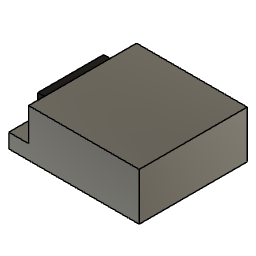
assembly_well plate track v43 (Autodesk Fusion 360 archive; units mm, degrees)
design "meanwell rd-35"
Autodesk Fusion 360 part; units mm, degrees
note: some values were not read from the file. Set by a fixed rule: the direction of a hole.
(part 1 of 2)
sketch "Sketch1" plane through (0, 0, 0) normal (0, 0, 1) x (1, 0, 0)
  line L0 (49.5, -41) -> (-49.5, -41)
  line L1 (-49.5, -41) -> (-49.5, 41)
  line L2 (-49.5, 41) -> (49.5, 41)
  line L3 (49.5, 41) -> (49.5, -41)
  line L4 (49.5, -41) -> (-49.5, 41) construction
  line L5 (-49.5, -41) -> (49.5, 41) construction
  line L6 (-29, -0.5) -> (26, -0.5)
  dimension "d1" = 99
  dimension "d2" = 82
  dimension "d3" = 40.5
  dimension "d4" = 20.5
  dimension "d5" = 55
  constraint horizontal L0
  constraint perpendicular L0 L1
  constraint parallel L0 L2
  constraint parallel L1 L3
  constraint coincident L4 origin
  constraint coincident L5 origin
  constraint horizontal L6
  measures "d1" distance of L1.end L2.end
  measures "d2" distance of L0.end L1.end
  measures "d3" distance of L0 L6
  measures "d4" distance of L1 L6.start
  measures "d5" distance of L6.start L6.end
extrude "Extrude1" add sketch "Sketch1" along normal blind 36 makes body 1
hole "Hole1" at (-29, -0.5, 0) at (26, -0.5, 0) direction (0, 0, 1) diameter 3 depth 10 tip angle 180 bodies 1
sketch "Sketch2" plane through (0, 0, 36) normal (0, 0, 1) x (-1, 0, 0)
  line L0 (-49.5, -41) -> (49.5, -41)
  line L1 (49.5, -41) -> (49.5, 41)
  line L2 (49.5, 41) -> (-49.5, 41)
  line L3 (-49.5, 41) -> (-49.5, -41)
  line L4 (49.5, -41) -> (34.5, -41)
  line L5 (34.5, -41) -> (34.5, 41)
  line L6 (34.5, 41) -> (49.5, 41)
  line L7 (49.5, 41) -> (49.5, -41)
  dimension "d11" = 15
  constraint horizontal L4
  constraint vertical L5
  constraint horizontal L6
  constraint vertical L7
  constraint coincident L2 L5.end
  constraint coincident L0.end L1.start
  measures "d11" distance of L0.end L4.end
extrude "Extrude2" cut sketch "Sketch2" against normal blind 25 contours L0 L1 L2 L4 L5 L6 L7 bodies 1
sketch "Sketch3" plane through (0, 0, 11) normal (0, 0, 1) x (-1, 0, 0)
  line L0 (49.5, 41) -> (34.5, 41)
  line L1 (34.5, 41) -> (34.5, -41)
  line L2 (34.5, -41) -> (49.5, -41)
  line L3 (49.5, -41) -> (49.5, 41)
  line L4 (49.5, -31) -> (34.5, -31)
  line L5 (34.5, -31) -> (34.5, 19)
  line L6 (34.5, 19) -> (49.5, 19)
  line L7 (49.5, 19) -> (49.5, -31)
  dimension "d14" = 10
  dimension "d15" = 50
  constraint horizontal L4
  constraint vertical L5
  constraint horizontal L6
  constraint vertical L7
  constraint coincident L1 L5.end
  constraint coincident L3 L4.start
  measures "d14" distance of L2 L4
  measures "d15" distance of L4.start L6.end
extrude "Extrude3" add sketch "Sketch3" along normal blind 15 separate body contours L1 L3 L4 L5 L6 L7 makes body 2

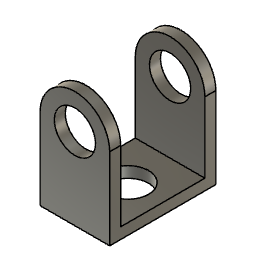
design "actuonix mounting bracket"
Autodesk Fusion 360 part; units mm, degrees
sketch "Sketch1" plane through (0, 0, 0) normal (0, 0, 1) x (1, 0, 0)
  line L0 (3.8, 5.8) -> (-3.8, 5.8)
  line L1 (-3.8, 5.8) -> (-3.8, -5.8)
  line L2 (-3.8, -5.8) -> (3.8, -5.8)
  line L3 (3.8, -5.8) -> (3.8, 5.8)
  line L4 (3.8, 5.8) -> (-3.8, -5.8) construction
  line L5 (-3.8, 5.8) -> (3.8, -5.8) construction
  dimension "d1" = 7.6
  dimension "d2" = 11.6
  constraint horizontal L0
  constraint perpendicular L0 L1
  constraint parallel L0 L2
  constraint parallel L1 L3
  constraint coincident L4 origin
  constraint coincident L5 origin
  measures "d1" distance of L0.start L0.end
  measures "d2" distance of L0.end L1.end
extrude "Extrude1" add sketch "Sketch1" along normal blind 12.7
sketch "Sketch2" plane through (3.8, 0, 0) normal (1, 0, 0) x (0, 1, 0)
  line L0 (-5.8, 0) -> (5.8, 0)
  line L1 (5.8, 0) -> (5.8, 12.7)
  line L2 (5.8, 12.7) -> (-5.8, 12.7)
  line L3 (-5.8, 12.7) -> (-5.8, 0)
  line L4 (-4.6, 11.5) -> (-4.6, 1.2)
  line L5 (-4.6, 1.2) -> (4.6, 1.2)
  line L6 (4.6, 1.2) -> (4.6, 11.5)
  line L7 (4.6, 11.5) -> (-4.6, 11.5)
  line L8 (4.6, 11.5) -> (4.6, 12.7)
  line L9 (-4.6, 11.5) -> (-4.6, 12.7)
  dimension "d5" = -1.2
  constraint coincident L2 L8.end
  constraint perpendicular L2 L8
  constraint coincident L2 L9.end
  constraint perpendicular L2 L9
extrude "Extrude2" cut sketch "Sketch2" against normal up to surface (7.6 mm away) contours L2 L7 L8 L9 | L4 L5 L6 L7
fillet "Fillet1" radius 3.8 4 edges at (3.8, 5.2, 12.7) (-3.8, 5.2, 12.7) (3.8, -5.2, 12.7) (-3.8, -5.2, 12.7)
hole "Hole1" at (0, 5.8, 8.9) direction (0, -1, 0) diameter 4.5 end through all
hole "Hole2" at (0, 0, 1.2) direction (0, 0, -1) diameter 4.5 end through all
equation "d9 = ( 7.6 / 2 ) * 1 mm"

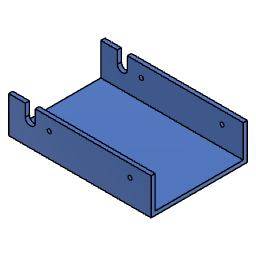
design "moving tray"
Autodesk Fusion 360 part; units mm, degrees
sketch "Sketch1" plane through (0, 0, 0) normal (0, 0, 1) x (1, 0, 0)
  line L0 (107.5, -72.5) -> (-107.5, -72.5)
  line L1 (-107.5, -72.5) -> (-107.5, 72.5)
  line L2 (-107.5, 72.5) -> (107.5, 72.5)
  line L3 (107.5, 72.5) -> (107.5, -72.5)
  line L4 (107.5, -72.5) -> (-107.5, 72.5) construction
  line L5 (-107.5, -72.5) -> (107.5, 72.5) construction
  dimension "d1" = 215
  dimension "d2" = 145
  constraint horizontal L0
  constraint perpendicular L0 L1
  constraint parallel L0 L2
  constraint parallel L1 L3
  constraint coincident L4 origin
  constraint coincident L5 origin
  measures "d1" distance of L1.end L2.end
  measures "d2" distance of L0.end L1.end
extrude "Extrude1" add sketch "Sketch1" along normal blind 55
sketch "Sketch2" plane through (-107.5, 0, 0) normal (-1, 0, 0) x (0, -1, 0)
  line L0 (-72.5, 0) -> (72.5, 0)
  line L1 (72.5, 0) -> (72.5, 55)
  line L2 (72.5, 55) -> (-72.5, 55)
  line L3 (-72.5, 55) -> (-72.5, 0)
  line L4 (-66.5, 49) -> (-66.5, 6)
  line L5 (-66.5, 6) -> (66.5, 6)
  line L6 (66.5, 6) -> (66.5, 49)
  line L7 (66.5, 49) -> (-66.5, 49)
  line L8 (66.5, 49) -> (66.5, 55)
  line L9 (-66.5, 49) -> (-66.5, 55)
  dimension "d5" = -6
  constraint coincident L2 L8.end
  constraint perpendicular L2 L8
  constraint coincident L2 L9.end
  constraint perpendicular L2 L9
extrude "Extrude2" cut sketch "Sketch2" against normal through all contours L2 L7 L8 L9 | L4 L5 L6 L7
sketch "Sketch3" plane through (0, 72.5, 0) normal (0, 1, 0) x (-1, 0, 0)
  line L0 (-107.5, 0) -> (107.5, 0)
  line L1 (107.5, 0) -> (107.5, 55)
  line L2 (107.5, 55) -> (-107.5, 55)
  line L3 (-107.5, 55) -> (-107.5, 0)
  line L4 (107.5, 6) -> (107.5, 55)
  line L5 (107.5, 36.5) -> (46.5, 36.5)
  line L6 (46.5, 36.5) -> (-75.5, 36.5)
  point P0 (46.5, 36.5)
  dimension "d7" = 122
  dimension "d8" = 61
  dimension "d9" = 18.5
  constraint perpendicular L1 L5
  constraint perpendicular L1 L6
  constraint coincident L4 L5.start
  constraint coincident P0 L5.end
  measures "d7" distance of P0 L6.end
  measures "d8" distance of L5.start P0
  measures "d9" distance of L2 L5
hole "Hole1" at (-46.5, 72.5, 36.5) at (75.5, 72.5, 36.5) direction (0, -1, 0) diameter 5.944 end through all
sketch "Sketch4" plane through (0, -72.5, 0) normal (0, -1, 0) x (1, 0, 0)
  circle A0 centre (-46.5, 36.5) radius 2.972
  circle A1 centre (75.5, 36.5) radius 2.972
  line L0 (-107.5, 0) -> (107.5, 0)
  line L1 (107.5, 0) -> (107.5, 55)
  line L2 (107.5, 55) -> (-107.5, 55)
  line L3 (-107.5, 55) -> (-107.5, 0)
  circle A2 centre (-75, 36.5) radius 7.5
  line L4 (-67.5, 36.5) -> (-67.5, 55)
  line L5 (-82.5, 36.5) -> (-82.5, 55)
  dimension "d13" = 28.5
  dimension "d14" = 15
  constraint horizontal A0.centre A2.centre
  constraint coincident A2 L4.start
  constraint coincident L2 L4.end
  constraint tangent A2 L4
  constraint coincident A2 L5.start
  constraint coincident L2 L5.end
  constraint tangent A2 L5
  constraint vertical L5
  constraint vertical L4
  measures "d13" distance of A0.centre A2.centre
  measures "d14" diameter of A2
extrude "Extrude3" cut sketch "Sketch4" against normal through all contours L2 A2 L4 L5 | A2

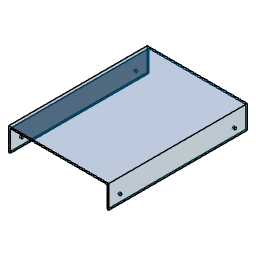
design "well plate base"
Autodesk Fusion 360 part; units mm, degrees
sketch "Sketch1" plane through (0, 0, 0) normal (0, 0, 1) x (1, 0, 0)
  line L0 (65, 90) -> (-65, 90)
  line L1 (-65, 90) -> (-65, -90)
  line L2 (-65, -90) -> (65, -90)
  line L3 (65, -90) -> (65, 90)
  line L4 (65, 90) -> (-65, -90) construction
  line L5 (-65, 90) -> (65, -90) construction
  dimension "d1" = 130
  dimension "d2" = 180
  constraint horizontal L0
  constraint perpendicular L0 L1
  constraint parallel L0 L2
  constraint parallel L1 L3
  constraint coincident L4 origin
  constraint coincident L5 origin
  measures "d1" distance of L1.end L2.end
  measures "d2" distance of L0.end L1.end
extrude "Extrude1" add sketch "Sketch1" along normal blind 30
shell "Shell1" thickness 2 removed faces 1 at (21.6667, -30, 0)
sketch "Sketch3" plane through (0, -90, 0) normal (0, -1, 0) x (1, 0, 0)
  line L0 (-65, 0) -> (65, 0)
  line L1 (65, 0) -> (65, 30)
  line L2 (65, 30) -> (-65, 30)
  line L3 (-65, 30) -> (-65, 0)
  line L4 (-63, 28) -> (63, 28)
  line L5 (63, 28) -> (63, 0)
  line L6 (63, 0) -> (-63, 0)
  line L7 (-63, 0) -> (-63, 28)
  point P0 (-63, 28)
  point P1 (63, 0)
  constraint horizontal L4
  constraint vertical L5
  constraint horizontal L6
  constraint vertical L7
  constraint coincident P1 L5.end
  constraint coincident P0 L4.start
extrude "Extrude3" cut sketch "Sketch3" against normal through all contours L0 L4 L5 L6 L7
sketch "Sketch4" plane through (65, 0, 0) normal (1, 0, 0) x (0, 1, 0)
  line L0 (-90, 0) -> (90, 0)
  line L1 (90, 0) -> (90, 30)
  line L2 (90, 30) -> (-90, 30)
  line L3 (-90, 30) -> (-90, 0)
  line L4 (-74.25, 10) -> (74.25, 10)
  line L5 (0, 0) -> (0, 10)
  dimension "d9" = 148.5
  dimension "d10" = 10
  constraint parallel L2 L4
  constraint coincident L5.start origin
  constraint coincident L4 L5.end
  constraint midpoint L4 L5.end
  constraint vertical L5
  measures "d9" distance of L4.start L4.end
  measures "d10" distance of L0 L4
hole "Hole1" at (65, -74.25, 10) at (65, 74.25, 10) direction (-1, 0, 0) diameter 3 depth 164 tip angle 118

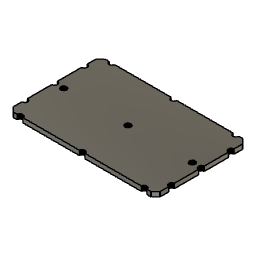
design "solderful protoboard"
Autodesk Fusion 360 part; units mm, degrees
sketch "SOLDERBREAD02_DXF_Outline_in_MilliMeters" plane through (0, 0, 0) normal (0, 0, 1) x (1, 0, 0)
  line L0 (116.847, -64.0665) -> (116.619, -64.1211)
  line L1 (116.619, -64.1211) -> (116.403, -64.2106)
  line L2 (116.403, -64.2106) -> (116.204, -64.3328)
  line L3 (116.204, -64.3328) -> (116.026, -64.4848)
  line L4 (116.026, -64.4848) -> (115.874, -64.6627)
  line L5 (115.874, -64.6627) -> (115.752, -64.8621)
  line L6 (115.752, -64.8621) -> (115.662, -65.0783)
  line L7 (115.662, -65.0783) -> (115.607, -65.3058)
  line L8 (115.607, -65.3058) -> (115.589, -65.539)
  line L9 (115.589, -65.539) -> (115.607, -65.7722)
  line L10 (115.607, -65.7722) -> (115.662, -65.9997)
  line L11 (115.662, -65.9997) -> (115.752, -66.2159)
  line L12 (115.752, -66.2159) -> (115.874, -66.4153)
  line L13 (115.874, -66.4153) -> (116.026, -66.5932)
  line L14 (116.026, -66.5932) -> (116.204, -66.7452)
  line L15 (116.204, -66.7452) -> (116.403, -66.8674)
  line L16 (116.403, -66.8674) -> (116.619, -66.9569)
  line L17 (116.619, -66.9569) -> (116.847, -67.0115)
  line L18 (116.847, -67.0115) -> (117.071, -67.0292)
  line L19 (117.071, -67.0292) -> (117.08, -67.0253)
  line L20 (117.08, -67.0253) -> (117.098, -67.0326)
  line L21 (117.098, -67.0326) -> (117.105, -67.0503)
  line L22 (117.105, -67.0503) -> (117.105, -80.511)
  line L23 (117.105, -80.511) -> (117.098, -80.5287)
  line L24 (117.098, -80.5287) -> (117.08, -80.536)
  line L25 (117.08, -80.536) -> (117.068, -80.531)
  line L26 (117.068, -80.531) -> (116.842, -80.5488)
  line L27 (116.842, -80.5488) -> (116.611, -80.6044)
  line L28 (116.611, -80.6044) -> (116.39, -80.6956)
  line L29 (116.39, -80.6956) -> (116.187, -80.8202)
  line L30 (116.187, -80.8202) -> (116.006, -80.975)
  line L31 (116.006, -80.975) -> (115.851, -81.1562)
  line L32 (115.851, -81.1562) -> (115.727, -81.3594)
  line L33 (115.727, -81.3594) -> (115.635, -81.5796)
  line L34 (115.635, -81.5796) -> (115.58, -81.8114)
  line L35 (115.58, -81.8114) -> (115.561, -82.049)
  line L36 (115.561, -82.049) -> (115.58, -82.2866)
  line L37 (115.58, -82.2866) -> (115.635, -82.5184)
  line L38 (115.635, -82.5184) -> (115.727, -82.7386)
  line L39 (115.727, -82.7386) -> (115.851, -82.9418)
  line L40 (115.851, -82.9418) -> (116.006, -83.123)
  line L41 (116.006, -83.123) -> (116.187, -83.2778)
  line L42 (116.187, -83.2778) -> (116.39, -83.4024)
  line L43 (116.39, -83.4024) -> (116.611, -83.4936)
  line L44 (116.611, -83.4936) -> (116.842, -83.5492)
  line L45 (116.842, -83.5492) -> (117.07, -83.5671)
  line L46 (117.07, -83.5671) -> (117.08, -83.563)
  line L47 (117.08, -83.563) -> (117.098, -83.5703)
  line L48 (117.098, -83.5703) -> (117.105, -83.588)
  line L49 (117.105, -83.588) -> (117.105, -88.233)
  line L50 (117.105, -88.233) -> (117.105, -88.2333)
  line L51 (117.105, -88.2333) -> (117.105, -88.2336)
  line L52 (117.105, -88.2336) -> (117.105, -88.2336)
  line L53 (117.105, -88.2336) -> (117.098, -88.3175)
  line L54 (117.098, -88.3175) -> (117.073, -88.3981)
  line L55 (117.073, -88.3981) -> (117.033, -88.4721)
  line L56 (117.033, -88.4721) -> (116.979, -88.535)
  line L57 (116.979, -88.535) -> (116.979, -88.5357)
  line L58 (116.979, -88.5357) -> (114.679, -90.8352)
  line L59 (114.679, -90.8352) -> (114.678, -90.8356)
  line L60 (114.678, -90.8356) -> (114.616, -90.8902)
  line L61 (114.616, -90.8902) -> (114.542, -90.9313)
  line L62 (114.542, -90.9313) -> (114.461, -90.9563)
  line L63 (114.461, -90.9563) -> (114.377, -90.964)
  line L64 (114.377, -90.964) -> (114.377, -90.964)
  line L65 (114.377, -90.964) -> (114.376, -90.9636)
  line L66 (114.376, -90.9636) -> (114.375, -90.964)
  line L67 (114.375, -90.964) -> (112.259, -90.964)
  line L68 (112.259, -90.964) -> (112.241, -90.9567)
  line L69 (112.241, -90.9567) -> (112.234, -90.939)
  line L70 (112.234, -90.939) -> (112.238, -90.9297)
  line L71 (112.238, -90.9297) -> (112.22, -90.7074)
  line L72 (112.22, -90.7074) -> (112.166, -90.4814)
  line L73 (112.166, -90.4814) -> (112.077, -90.2668)
  line L74 (112.077, -90.2668) -> (111.956, -90.0687)
  line L75 (111.956, -90.0687) -> (111.805, -89.892)
  line L76 (111.805, -89.892) -> (111.628, -89.7411)
  line L77 (111.628, -89.7411) -> (111.43, -89.6197)
  line L78 (111.43, -89.6197) -> (111.216, -89.5308)
  line L79 (111.216, -89.5308) -> (110.99, -89.4765)
  line L80 (110.99, -89.4765) -> (110.758, -89.4583)
  line L81 (110.758, -89.4583) -> (110.526, -89.4765)
  line L82 (110.526, -89.4765) -> (110.3, -89.5308)
  line L83 (110.3, -89.5308) -> (110.086, -89.6197)
  line L84 (110.086, -89.6197) -> (109.888, -89.7411)
  line L85 (109.888, -89.7411) -> (109.711, -89.892)
  line L86 (109.711, -89.892) -> (109.56, -90.0687)
  line L87 (109.56, -90.0687) -> (109.439, -90.2668)
  line L88 (109.439, -90.2668) -> (109.35, -90.4814)
  line L89 (109.35, -90.4814) -> (109.295, -90.7074)
  line L90 (109.295, -90.7074) -> (109.278, -90.9297)
  line L91 (109.278, -90.9297) -> (109.282, -90.939)
  line L92 (109.282, -90.939) -> (109.274, -90.9567)
  line L93 (109.274, -90.9567) -> (109.257, -90.964)
  line L94 (109.257, -90.964) -> (77.964, -90.964)
  line L95 (77.964, -90.964) -> (77.9463, -90.9567)
  line L96 (77.9463, -90.9567) -> (77.939, -90.939)
  line L97 (77.939, -90.939) -> (77.9429, -90.9296)
  line L98 (77.9429, -90.9296) -> (77.9251, -90.7038)
  line L99 (77.9251, -90.7038) -> (77.87, -90.4744)
  line L100 (77.87, -90.4744) -> (77.7797, -90.2564)
  line L101 (77.7797, -90.2564) -> (77.6565, -90.0552)
  line L102 (77.6565, -90.0552) -> (77.5032, -89.8758)
  line L103 (77.5032, -89.8758) -> (77.3238, -89.7225)
  line L104 (77.3238, -89.7225) -> (77.1226, -89.5993)
  line L105 (77.1226, -89.5993) -> (76.9046, -89.509)
  line L106 (76.9046, -89.509) -> (76.6752, -89.4539)
  line L107 (76.6752, -89.4539) -> (76.44, -89.4354)
  line L108 (76.44, -89.4354) -> (76.2048, -89.4539)
  line L109 (76.2048, -89.4539) -> (75.9754, -89.509)
  line L110 (75.9754, -89.509) -> (75.7574, -89.5993)
  line L111 (75.7574, -89.5993) -> (75.5562, -89.7225)
  line L112 (75.5562, -89.7225) -> (75.3768, -89.8758)
  line L113 (75.3768, -89.8758) -> (75.2235, -90.0552)
  line L114 (75.2235, -90.0552) -> (75.1003, -90.2564)
  line L115 (75.1003, -90.2564) -> (75.01, -90.4744)
  line L116 (75.01, -90.4744) -> (74.9549, -90.7038)
  line L117 (74.9549, -90.7038) -> (74.9371, -90.9296)
  line L118 (74.9371, -90.9296) -> (74.941, -90.939)
  line L119 (74.941, -90.939) -> (74.9337, -90.9567)
  line L120 (74.9337, -90.9567) -> (74.916, -90.964)
  line L121 (74.916, -90.964) -> (43.6638, -90.964)
  line L122 (43.6638, -90.964) -> (43.6462, -90.9567)
  line L123 (43.6462, -90.9567) -> (43.6388, -90.939)
  line L124 (43.6388, -90.939) -> (43.6392, -90.9382)
  line L125 (43.6392, -90.9382) -> (43.6428, -90.9295)
  line L126 (43.6428, -90.9295) -> (43.6248, -90.7014)
  line L127 (43.6248, -90.7014) -> (43.5692, -90.4696)
  line L128 (43.5692, -90.4696) -> (43.478, -90.2494)
  line L129 (43.478, -90.2494) -> (43.3534, -90.0462)
  line L130 (43.3534, -90.0462) -> (43.1986, -89.865)
  line L131 (43.1986, -89.865) -> (43.0174, -89.7102)
  line L132 (43.0174, -89.7102) -> (42.8142, -89.5856)
  line L133 (42.8142, -89.5856) -> (42.594, -89.4944)
  line L134 (42.594, -89.4944) -> (42.3622, -89.4388)
  line L135 (42.3622, -89.4388) -> (42.1246, -89.4201)
  line L136 (42.1246, -89.4201) -> (41.887, -89.4388)
  line L137 (41.887, -89.4388) -> (41.6552, -89.4944)
  line L138 (41.6552, -89.4944) -> (41.435, -89.5856)
  line L139 (41.435, -89.5856) -> (41.2318, -89.7102)
  line L140 (41.2318, -89.7102) -> (41.0506, -89.865)
  line L141 (41.0506, -89.865) -> (40.8958, -90.0462)
  line L142 (40.8958, -90.0462) -> (40.7712, -90.2494)
  line L143 (40.7712, -90.2494) -> (40.68, -90.4696)
  line L144 (40.68, -90.4696) -> (40.6244, -90.7014)
  line L145 (40.6244, -90.7014) -> (40.6064, -90.9295)
  line L146 (40.6064, -90.9295) -> (40.61, -90.9382)
  line L147 (40.61, -90.9382) -> (40.6104, -90.939)
  line L148 (40.6104, -90.939) -> (40.603, -90.9567)
  line L149 (40.603, -90.9567) -> (40.5854, -90.964)
  line L150 (40.5854, -90.964) -> (38.509, -90.964)
  line L151 (38.509, -90.964) -> (38.5088, -90.9639)
  line L152 (38.5088, -90.9639) -> (38.4247, -90.9577)
  line L153 (38.4247, -90.9577) -> (38.3428, -90.9337)
  line L154 (38.3428, -90.9337) -> (38.2677, -90.8931)
  line L155 (38.2677, -90.8931) -> (38.2028, -90.8376)
  line L156 (38.2028, -90.8376) -> (38.2029, -90.8376)
  line L157 (38.2029, -90.8376) -> (38.2026, -90.837)
  line L158 (38.2026, -90.837) -> (35.902, -88.5364)
  line L159 (35.902, -88.5364) -> (35.9014, -88.5361)
  line L160 (35.9014, -88.5361) -> (35.846, -88.4713)
  line L161 (35.846, -88.4713) -> (35.8053, -88.3962)
  line L162 (35.8053, -88.3962) -> (35.7813, -88.3143)
  line L163 (35.7813, -88.3143) -> (35.775, -88.2293)
  line L164 (35.775, -88.2293) -> (35.775, -88.2292)
  line L165 (35.775, -88.2292) -> (35.7753, -88.2286)
  line L166 (35.7753, -88.2286) -> (35.775, -88.228)
  line L167 (35.775, -88.228) -> (35.775, -83.589)
  line L168 (35.775, -83.589) -> (35.7752, -83.5886)
  line L169 (35.7752, -83.5886) -> (35.775, -83.5882)
  line L170 (35.775, -83.5882) -> (35.7823, -83.5706)
  line L171 (35.7823, -83.5706) -> (35.8, -83.5632)
  line L172 (35.8, -83.5632) -> (35.8095, -83.5672)
  line L173 (35.8095, -83.5672) -> (36.0376, -83.5492)
  line L174 (36.0376, -83.5492) -> (36.2694, -83.4936)
  line L175 (36.2694, -83.4936) -> (36.4896, -83.4024)
  line L176 (36.4896, -83.4024) -> (36.6928, -83.2778)
  line L177 (36.6928, -83.2778) -> (36.874, -83.123)
  line L178 (36.874, -83.123) -> (37.0288, -82.9418)
  line L179 (37.0288, -82.9418) -> (37.1534, -82.7386)
  line L180 (37.1534, -82.7386) -> (37.2446, -82.5184)
  line L181 (37.2446, -82.5184) -> (37.3002, -82.2866)
  line L182 (37.3002, -82.2866) -> (37.3189, -82.049)
  line L183 (37.3189, -82.049) -> (37.3002, -81.8114)
  line L184 (37.3002, -81.8114) -> (37.2446, -81.5796)
  line L185 (37.2446, -81.5796) -> (37.1534, -81.3594)
  line L186 (37.1534, -81.3594) -> (37.0288, -81.1562)
  line L187 (37.0288, -81.1562) -> (36.874, -80.975)
  line L188 (36.874, -80.975) -> (36.6928, -80.8202)
  line L189 (36.6928, -80.8202) -> (36.4896, -80.6956)
  line L190 (36.4896, -80.6956) -> (36.2694, -80.6044)
  line L191 (36.2694, -80.6044) -> (36.0376, -80.5488)
  line L192 (36.0376, -80.5488) -> (35.8095, -80.5308)
  line L193 (35.8095, -80.5308) -> (35.8, -80.5348)
  line L194 (35.8, -80.5348) -> (35.7823, -80.5274)
  line L195 (35.7823, -80.5274) -> (35.775, -80.5098)
  line L196 (35.775, -80.5098) -> (35.7756, -80.5084)
  line L197 (35.7756, -80.5084) -> (35.775, -80.507)
  line L198 (35.775, -80.507) -> (35.775, -67.0605)
  line L199 (35.775, -67.0605) -> (35.7823, -67.0428)
  line L200 (35.7823, -67.0428) -> (35.8, -67.0355)
  line L201 (35.8, -67.0355) -> (35.8094, -67.0393)
  line L202 (35.8094, -67.0393) -> (36.0348, -67.0216)
  line L203 (36.0348, -67.0216) -> (36.2639, -66.9666)
  line L204 (36.2639, -66.9666) -> (36.4815, -66.8765)
  line L205 (36.4815, -66.8765) -> (36.6823, -66.7534)
  line L206 (36.6823, -66.7534) -> (36.8614, -66.6004)
  line L207 (36.8614, -66.6004) -> (37.0144, -66.4213)
  line L208 (37.0144, -66.4213) -> (37.1375, -66.2205)
  line L209 (37.1375, -66.2205) -> (37.2276, -66.0029)
  line L210 (37.2276, -66.0029) -> (37.2826, -65.7738)
  line L211 (37.2826, -65.7738) -> (37.3011, -65.539)
  line L212 (37.3011, -65.539) -> (37.2826, -65.3042)
  line L213 (37.2826, -65.3042) -> (37.2276, -65.0751)
  line L214 (37.2276, -65.0751) -> (37.1375, -64.8575)
  line L215 (37.1375, -64.8575) -> (37.0144, -64.6567)
  line L216 (37.0144, -64.6567) -> (36.8614, -64.4776)
  line L217 (36.8614, -64.4776) -> (36.6823, -64.3246)
  line L218 (36.6823, -64.3246) -> (36.4815, -64.2015)
  line L219 (36.4815, -64.2015) -> (36.2639, -64.1114)
  line L220 (36.2639, -64.1114) -> (36.0348, -64.0564)
  line L221 (36.0348, -64.0564) -> (35.8094, -64.0387)
  line L222 (35.8094, -64.0387) -> (35.8, -64.0425)
  line L223 (35.8, -64.0425) -> (35.7823, -64.0352)
  line L224 (35.7823, -64.0352) -> (35.775, -64.0175)
  line L225 (35.775, -64.0175) -> (35.775, -50.568)
  line L226 (35.775, -50.568) -> (35.7823, -50.5503)
  line L227 (35.7823, -50.5503) -> (35.8, -50.543)
  line L228 (35.8, -50.543) -> (35.81, -50.5471)
  line L229 (35.81, -50.5471) -> (36.0376, -50.5292)
  line L230 (36.0376, -50.5292) -> (36.2694, -50.4736)
  line L231 (36.2694, -50.4736) -> (36.4896, -50.3824)
  line L232 (36.4896, -50.3824) -> (36.6928, -50.2578)
  line L233 (36.6928, -50.2578) -> (36.874, -50.103)
  line L234 (36.874, -50.103) -> (37.0288, -49.9218)
  line L235 (37.0288, -49.9218) -> (37.1534, -49.7186)
  line L236 (37.1534, -49.7186) -> (37.2446, -49.4984)
  line L237 (37.2446, -49.4984) -> (37.3002, -49.2666)
  line L238 (37.3002, -49.2666) -> (37.3189, -49.029)
  line L239 (37.3189, -49.029) -> (37.3002, -48.7914)
  line L240 (37.3002, -48.7914) -> (37.2446, -48.5596)
  line L241 (37.2446, -48.5596) -> (37.1534, -48.3394)
  line L242 (37.1534, -48.3394) -> (37.0288, -48.1362)
  line L243 (37.0288, -48.1362) -> (36.874, -47.955)
  line L244 (36.874, -47.955) -> (36.6928, -47.8002)
  line L245 (36.6928, -47.8002) -> (36.4896, -47.6756)
  line L246 (36.4896, -47.6756) -> (36.2694, -47.5844)
  line L247 (36.2694, -47.5844) -> (36.0376, -47.5288)
  line L248 (36.0376, -47.5288) -> (35.8095, -47.5108)
  line L249 (35.8095, -47.5108) -> (35.8, -47.5148)
  line L250 (35.8, -47.5148) -> (35.7823, -47.5074)
  line L251 (35.7823, -47.5074) -> (35.775, -47.4898)
  line L252 (35.775, -47.4898) -> (35.7756, -47.4884)
  line L253 (35.7756, -47.4884) -> (35.775, -47.487)
  line L254 (35.775, -47.487) -> (35.775, -42.836)
  line L255 (35.775, -42.836) -> (35.7752, -42.8356)
  line L256 (35.7752, -42.8356) -> (35.7831, -42.7565)
  line L257 (35.7831, -42.7565) -> (35.8069, -42.6792)
  line L258 (35.8069, -42.6792) -> (35.8456, -42.6081)
  line L259 (35.8456, -42.6081) -> (35.8973, -42.5464)
  line L260 (35.8973, -42.5464) -> (35.8973, -42.5463)
  line L261 (35.8973, -42.5463) -> (38.2026, -40.241)
  line L262 (38.2026, -40.241) -> (38.2028, -40.2404)
  line L263 (38.2028, -40.2404) -> (38.2028, -40.2404)
  line L264 (38.2028, -40.2404) -> (38.2677, -40.185)
  line L265 (38.2677, -40.185) -> (38.3428, -40.1443)
  line L266 (38.3428, -40.1443) -> (38.4247, -40.1203)
  line L267 (38.4247, -40.1203) -> (38.5087, -40.1141)
  line L268 (38.5087, -40.1141) -> (38.509, -40.114)
  line L269 (38.509, -40.114) -> (40.7073, -40.114)
  line L270 (40.7073, -40.114) -> (40.725, -40.1213)
  line L271 (40.725, -40.1213) -> (40.7323, -40.139)
  line L272 (40.7323, -40.139) -> (40.7301, -40.1443)
  line L273 (40.7301, -40.1443) -> (40.7287, -40.1477)
  line L274 (40.7287, -40.1477) -> (40.7452, -40.3575)
  line L275 (40.7452, -40.3575) -> (40.7963, -40.5706)
  line L276 (40.7963, -40.5706) -> (40.8802, -40.7731)
  line L277 (40.8802, -40.7731) -> (40.9947, -40.9599)
  line L278 (40.9947, -40.9599) -> (41.137, -41.1266)
  line L279 (41.137, -41.1266) -> (41.3037, -41.2689)
  line L280 (41.3037, -41.2689) -> (41.4905, -41.3834)
  line L281 (41.4905, -41.3834) -> (41.693, -41.4673)
  line L282 (41.693, -41.4673) -> (41.9061, -41.5184)
  line L283 (41.9061, -41.5184) -> (42.1246, -41.5356)
  line L284 (42.1246, -41.5356) -> (42.3431, -41.5184)
  line L285 (42.3431, -41.5184) -> (42.5562, -41.4673)
  line L286 (42.5562, -41.4673) -> (42.7587, -41.3834)
  line L287 (42.7587, -41.3834) -> (42.9455, -41.2689)
  line L288 (42.9455, -41.2689) -> (43.1122, -41.1266)
  line L289 (43.1122, -41.1266) -> (43.2545, -40.9599)
  line L290 (43.2545, -40.9599) -> (43.369, -40.7731)
  line L291 (43.369, -40.7731) -> (43.4529, -40.5706)
  line L292 (43.4529, -40.5706) -> (43.504, -40.3575)
  line L293 (43.504, -40.3575) -> (43.5205, -40.1477)
  line L294 (43.5205, -40.1477) -> (43.5191, -40.1443)
  line L295 (43.5191, -40.1443) -> (43.5169, -40.139)
  line L296 (43.5169, -40.139) -> (43.5242, -40.1213)
  line L297 (43.5242, -40.1213) -> (43.5419, -40.114)
  line L298 (43.5419, -40.114) -> (74.916, -40.114)
  line L299 (74.916, -40.114) -> (74.9337, -40.1213)
  line L300 (74.9337, -40.1213) -> (74.941, -40.139)
  line L301 (74.941, -40.139) -> (74.9371, -40.1484)
  line L302 (74.9371, -40.1484) -> (74.9549, -40.3742)
  line L303 (74.9549, -40.3742) -> (75.01, -40.6036)
  line L304 (75.01, -40.6036) -> (75.1003, -40.8216)
  line L305 (75.1003, -40.8216) -> (75.2235, -41.0228)
  line L306 (75.2235, -41.0228) -> (75.3768, -41.2022)
  line L307 (75.3768, -41.2022) -> (75.5562, -41.3555)
  line L308 (75.5562, -41.3555) -> (75.7574, -41.4787)
  line L309 (75.7574, -41.4787) -> (75.9754, -41.569)
  line L310 (75.9754, -41.569) -> (76.2048, -41.6241)
  line L311 (76.2048, -41.6241) -> (76.44, -41.6426)
  line L312 (76.44, -41.6426) -> (76.6752, -41.6241)
  line L313 (76.6752, -41.6241) -> (76.9046, -41.569)
  line L314 (76.9046, -41.569) -> (77.1226, -41.4787)
  line L315 (77.1226, -41.4787) -> (77.3238, -41.3555)
  line L316 (77.3238, -41.3555) -> (77.5032, -41.2022)
  line L317 (77.5032, -41.2022) -> (77.6565, -41.0228)
  line L318 (77.6565, -41.0228) -> (77.7797, -40.8216)
  line L319 (77.7797, -40.8216) -> (77.87, -40.6036)
  line L320 (77.87, -40.6036) -> (77.9251, -40.3742)
  line L321 (77.9251, -40.3742) -> (77.9429, -40.1484)
  line L322 (77.9429, -40.1484) -> (77.939, -40.139)
  line L323 (77.939, -40.139) -> (77.9463, -40.1213)
  line L324 (77.9463, -40.1213) -> (77.964, -40.114)
  line L325 (77.964, -40.114) -> (109.257, -40.114)
  line L326 (109.257, -40.114) -> (109.258, -40.1145)
  line L327 (109.258, -40.1145) -> (109.259, -40.114)
  line L328 (109.259, -40.114) -> (109.277, -40.1214)
  line L329 (109.277, -40.1214) -> (109.284, -40.139)
  line L330 (109.284, -40.139) -> (109.28, -40.1484)
  line L331 (109.28, -40.1484) -> (109.298, -40.3706)
  line L332 (109.298, -40.3706) -> (109.351, -40.5964)
  line L333 (109.351, -40.5964) -> (109.44, -40.8111)
  line L334 (109.44, -40.8111) -> (109.561, -41.0092)
  line L335 (109.561, -41.0092) -> (109.712, -41.1859)
  line L336 (109.712, -41.1859) -> (109.888, -41.3368)
  line L337 (109.888, -41.3368) -> (110.086, -41.4582)
  line L338 (110.086, -41.4582) -> (110.301, -41.5472)
  line L339 (110.301, -41.5472) -> (110.526, -41.6015)
  line L340 (110.526, -41.6015) -> (110.758, -41.6197)
  line L341 (110.758, -41.6197) -> (110.989, -41.6015)
  line L342 (110.989, -41.6015) -> (111.215, -41.5472)
  line L343 (111.215, -41.5472) -> (111.43, -41.4582)
  line L344 (111.43, -41.4582) -> (111.628, -41.3368)
  line L345 (111.628, -41.3368) -> (111.804, -41.1859)
  line L346 (111.804, -41.1859) -> (111.955, -41.0092)
  line L347 (111.955, -41.0092) -> (112.076, -40.811)
  line L348 (112.076, -40.811) -> (112.164, -40.5964)
  line L349 (112.164, -40.5964) -> (112.218, -40.3705)
  line L350 (112.218, -40.3705) -> (112.235, -40.1483)
  line L351 (112.235, -40.1483) -> (112.232, -40.139)
  line L352 (112.232, -40.139) -> (112.232, -40.139)
  line L353 (112.232, -40.139) -> (112.232, -40.139)
  line L354 (112.232, -40.139) -> (112.235, -40.1307)
  line L355 (112.235, -40.1307) -> (112.239, -40.1214)
  line L356 (112.239, -40.1214) -> (112.239, -40.1213)
  line L357 (112.239, -40.1213) -> (112.239, -40.1213)
  line L358 (112.239, -40.1213) -> (112.247, -40.1179)
  line L359 (112.247, -40.1179) -> (112.256, -40.114)
  line L360 (112.256, -40.114) -> (112.257, -40.114)
  line L361 (112.257, -40.114) -> (112.257, -40.114)
  line L362 (112.257, -40.114) -> (114.371, -40.114)
  line L363 (114.371, -40.114) -> (114.371, -40.1141)
  line L364 (114.371, -40.1141) -> (114.455, -40.1203)
  line L365 (114.455, -40.1203) -> (114.537, -40.1443)
  line L366 (114.537, -40.1443) -> (114.612, -40.1849)
  line L367 (114.612, -40.1849) -> (114.677, -40.2404)
  line L368 (114.677, -40.2404) -> (114.677, -40.2404)
  line L369 (114.677, -40.2404) -> (114.677, -40.241)
  line L370 (114.677, -40.241) -> (116.979, -42.5428)
  line L371 (116.979, -42.5428) -> (116.98, -42.5442)
  line L372 (116.98, -42.5442) -> (117.034, -42.6077)
  line L373 (117.034, -42.6077) -> (117.075, -42.6828)
  line L374 (117.075, -42.6828) -> (117.099, -42.7647)
  line L375 (117.099, -42.7647) -> (117.105, -42.8451)
  line L376 (117.105, -42.8451) -> (117.105, -42.846)
  line L377 (117.105, -42.846) -> (117.105, -47.489)
  line L378 (117.105, -47.489) -> (117.105, -47.4894)
  line L379 (117.105, -47.4894) -> (117.105, -47.4898)
  line L380 (117.105, -47.4898) -> (117.098, -47.5074)
  line L381 (117.098, -47.5074) -> (117.08, -47.5148)
  line L382 (117.08, -47.5148) -> (117.071, -47.5108)
  line L383 (117.071, -47.5108) -> (116.842, -47.5288)
  line L384 (116.842, -47.5288) -> (116.611, -47.5844)
  line L385 (116.611, -47.5844) -> (116.39, -47.6756)
  line L386 (116.39, -47.6756) -> (116.187, -47.8002)
  line L387 (116.187, -47.8002) -> (116.006, -47.955)
  line L388 (116.006, -47.955) -> (115.851, -48.1362)
  line L389 (115.851, -48.1362) -> (115.727, -48.3394)
  line L390 (115.727, -48.3394) -> (115.635, -48.5596)
  line L391 (115.635, -48.5596) -> (115.58, -48.7914)
  line L392 (115.58, -48.7914) -> (115.561, -49.029)
  line L393 (115.561, -49.029) -> (115.58, -49.2666)
  line L394 (115.58, -49.2666) -> (115.635, -49.4984)
  line L395 (115.635, -49.4984) -> (115.727, -49.7186)
  line L396 (115.727, -49.7186) -> (115.851, -49.9218)
  line L397 (115.851, -49.9218) -> (116.006, -50.103)
  line L398 (116.006, -50.103) -> (116.187, -50.2578)
  line L399 (116.187, -50.2578) -> (116.39, -50.3824)
  line L400 (116.39, -50.3824) -> (116.611, -50.4736)
  line L401 (116.611, -50.4736) -> (116.842, -50.5292)
  line L402 (116.842, -50.5292) -> (117.071, -50.5472)
  line L403 (117.071, -50.5472) -> (117.08, -50.5432)
  line L404 (117.08, -50.5432) -> (117.098, -50.5506)
  line L405 (117.098, -50.5506) -> (117.105, -50.5682)
  line L406 (117.105, -50.5682) -> (117.105, -64.0277)
  line L407 (117.105, -64.0277) -> (117.098, -64.0454)
  line L408 (117.098, -64.0454) -> (117.08, -64.0527)
  line L409 (117.08, -64.0527) -> (117.071, -64.0488)
  line L410 (117.071, -64.0488) -> (116.847, -64.0665)
  line L411 (109.251, -90.7003) -> (109.306, -90.4674)
  line L412 (109.306, -90.4674) -> (109.398, -90.2461)
  line L413 (109.398, -90.2461) -> (109.523, -90.042)
  line L414 (109.523, -90.042) -> (109.679, -89.8599)
  line L415 (109.679, -89.8599) -> (109.861, -89.7043)
  line L416 (109.861, -89.7043) -> (110.065, -89.5792)
  line L417 (110.065, -89.5792) -> (110.286, -89.4876)
  line L418 (110.286, -89.4876) -> (110.519, -89.4316)
  line L419 (110.519, -89.4316) -> (110.758, -89.4129)
  line L420 (110.758, -89.4129) -> (110.997, -89.4316)
  line L421 (110.997, -89.4316) -> (111.23, -89.4876)
  line L422 (111.23, -89.4876) -> (111.451, -89.5792)
  line L423 (111.451, -89.5792) -> (111.655, -89.7043)
  line L424 (111.655, -89.7043) -> (111.837, -89.8599)
  line L425 (111.837, -89.8599) -> (111.993, -90.042)
  line L426 (111.993, -90.042) -> (112.118, -90.2461)
  line L427 (112.118, -90.2461) -> (112.209, -90.4674)
  line L428 (112.209, -90.4674) -> (112.265, -90.7003)
  line L429 (112.265, -90.7003) -> (112.282, -90.914)
  line L430 (112.282, -90.914) -> (114.375, -90.914)
  line L431 (114.375, -90.914) -> (114.376, -90.9145)
  line L432 (114.376, -90.9145) -> (114.377, -90.914)
  line L433 (114.377, -90.914) -> (114.383, -90.9166)
  line L434 (114.383, -90.9166) -> (114.476, -90.9048)
  line L435 (114.476, -90.9048) -> (114.568, -90.8657)
  line L436 (114.568, -90.8657) -> (114.64, -90.8067)
  line L437 (114.64, -90.8067) -> (114.643, -90.8006)
  line L438 (114.643, -90.8006) -> (114.644, -90.8001)
  line L439 (114.644, -90.8001) -> (114.644, -90.7998)
  line L440 (114.644, -90.7998) -> (116.943, -88.5003)
  line L441 (116.943, -88.5003) -> (116.943, -88.5003)
  line L442 (116.943, -88.5003) -> (116.944, -88.4999)
  line L443 (116.944, -88.4999) -> (116.95, -88.4975)
  line L444 (116.95, -88.4975) -> (117.008, -88.4246)
  line L445 (117.008, -88.4246) -> (117.046, -88.3329)
  line L446 (117.046, -88.3329) -> (117.058, -88.2404)
  line L447 (117.058, -88.2404) -> (117.055, -88.2343)
  line L448 (117.055, -88.2343) -> (117.055, -88.2337)
  line L449 (117.055, -88.2337) -> (117.055, -88.233)
  line L450 (117.055, -88.233) -> (117.055, -83.6114)
  line L451 (117.055, -83.6114) -> (116.847, -83.5958)
  line L452 (116.847, -83.5958) -> (116.619, -83.5437)
  line L453 (116.619, -83.5437) -> (116.401, -83.4583)
  line L454 (116.401, -83.4583) -> (116.199, -83.3414)
  line L455 (116.199, -83.3414) -> (116.016, -83.1957)
  line L456 (116.016, -83.1957) -> (115.857, -83.0243)
  line L457 (115.857, -83.0243) -> (115.725, -82.8311)
  line L458 (115.725, -82.8311) -> (115.624, -82.6205)
  line L459 (115.624, -82.6205) -> (115.555, -82.3971)
  line L460 (115.555, -82.3971) -> (115.52, -82.1659)
  line L461 (115.52, -82.1659) -> (115.52, -81.9321)
  line L462 (115.52, -81.9321) -> (115.555, -81.7009)
  line L463 (115.555, -81.7009) -> (115.624, -81.4775)
  line L464 (115.624, -81.4775) -> (115.725, -81.2669)
  line L465 (115.725, -81.2669) -> (115.857, -81.0737)
  line L466 (115.857, -81.0737) -> (116.016, -80.9023)
  line L467 (116.016, -80.9023) -> (116.199, -80.7566)
  line L468 (116.199, -80.7566) -> (116.401, -80.6397)
  line L469 (116.401, -80.6397) -> (116.619, -80.5543)
  line L470 (116.619, -80.5543) -> (116.847, -80.5022)
  line L471 (116.847, -80.5022) -> (117.055, -80.4866)
  line L472 (117.055, -80.4866) -> (117.055, -67.0733)
  line L473 (117.055, -67.0733) -> (116.84, -67.0564)
  line L474 (116.84, -67.0564) -> (116.605, -67.0001)
  line L475 (116.605, -67.0001) -> (116.383, -66.9079)
  line L476 (116.383, -66.9079) -> (116.177, -66.7819)
  line L477 (116.177, -66.7819) -> (115.994, -66.6253)
  line L478 (115.994, -66.6253) -> (115.837, -66.442)
  line L479 (115.837, -66.442) -> (115.711, -66.2365)
  line L480 (115.711, -66.2365) -> (115.619, -66.0137)
  line L481 (115.619, -66.0137) -> (115.563, -65.7793)
  line L482 (115.563, -65.7793) -> (115.544, -65.539)
  line L483 (115.544, -65.539) -> (115.563, -65.2987)
  line L484 (115.563, -65.2987) -> (115.619, -65.0643)
  line L485 (115.619, -65.0643) -> (115.711, -64.8415)
  line L486 (115.711, -64.8415) -> (115.837, -64.636)
  line L487 (115.837, -64.636) -> (115.994, -64.4527)
  line L488 (115.994, -64.4527) -> (116.177, -64.2961)
  line L489 (116.177, -64.2961) -> (116.383, -64.1701)
  line L490 (116.383, -64.1701) -> (116.605, -64.0779)
  line L491 (116.605, -64.0779) -> (116.84, -64.0216)
  line L492 (116.84, -64.0216) -> (117.055, -64.0047)
  line L493 (117.055, -64.0047) -> (117.055, -50.5914)
  line L494 (117.055, -50.5914) -> (116.847, -50.5758)
  line L495 (116.847, -50.5758) -> (116.619, -50.5237)
  line L496 (116.619, -50.5237) -> (116.401, -50.4383)
  line L497 (116.401, -50.4383) -> (116.199, -50.3214)
  line L498 (116.199, -50.3214) -> (116.016, -50.1757)
  line L499 (116.016, -50.1757) -> (115.857, -50.0043)
  line L500 (115.857, -50.0043) -> (115.725, -49.8111)
  line L501 (115.725, -49.8111) -> (115.624, -49.6005)
  line L502 (115.624, -49.6005) -> (115.555, -49.3771)
  line L503 (115.555, -49.3771) -> (115.52, -49.1459)
  line L504 (115.52, -49.1459) -> (115.52, -48.9121)
  line L505 (115.52, -48.9121) -> (115.555, -48.6809)
  line L506 (115.555, -48.6809) -> (115.624, -48.4575)
  line L507 (115.624, -48.4575) -> (115.725, -48.2469)
  line L508 (115.725, -48.2469) -> (115.857, -48.0537)
  line L509 (115.857, -48.0537) -> (116.016, -47.8823)
  line L510 (116.016, -47.8823) -> (116.199, -47.7366)
  line L511 (116.199, -47.7366) -> (116.401, -47.6197)
  line L512 (116.401, -47.6197) -> (116.619, -47.5343)
  line L513 (116.619, -47.5343) -> (116.847, -47.4822)
  line L514 (116.847, -47.4822) -> (117.055, -47.4666)
  line L515 (117.055, -47.4666) -> (117.055, -42.846)
  line L516 (117.055, -42.846) -> (117.057, -42.8424)
  line L517 (117.057, -42.8424) -> (117.051, -42.7733)
  line L518 (117.051, -42.7733) -> (117.03, -42.7011)
  line L519 (117.03, -42.7011) -> (116.994, -42.6349)
  line L520 (116.994, -42.6349) -> (116.948, -42.5806)
  line L521 (116.948, -42.5806) -> (116.944, -42.5792)
  line L522 (116.944, -42.5792) -> (116.944, -42.5781)
  line L523 (116.944, -42.5781) -> (114.64, -40.2742)
  line L524 (114.64, -40.2742) -> (114.638, -40.2698)
  line L525 (114.638, -40.2698) -> (114.585, -40.2246)
  line L526 (114.585, -40.2246) -> (114.519, -40.1887)
  line L527 (114.519, -40.1887) -> (114.447, -40.1676)
  line L528 (114.447, -40.1676) -> (114.376, -40.1623)
  line L529 (114.376, -40.1623) -> (114.372, -40.164)
  line L530 (114.372, -40.164) -> (114.371, -40.1638)
  line L531 (114.371, -40.1638) -> (114.371, -40.164)
  line L532 (114.371, -40.164) -> (112.28, -40.164)
  line L533 (112.28, -40.164) -> (112.263, -40.3776)
  line L534 (112.263, -40.3776) -> (112.208, -40.6104)
  line L535 (112.208, -40.6104) -> (112.116, -40.8316)
  line L536 (112.116, -40.8316) -> (111.991, -41.0358)
  line L537 (111.991, -41.0358) -> (111.836, -41.218)
  line L538 (111.836, -41.218) -> (111.654, -41.3736)
  line L539 (111.654, -41.3736) -> (111.45, -41.4987)
  line L540 (111.45, -41.4987) -> (111.229, -41.5904)
  line L541 (111.229, -41.5904) -> (110.997, -41.6463)
  line L542 (110.997, -41.6463) -> (110.758, -41.6651)
  line L543 (110.758, -41.6651) -> (110.519, -41.6463)
  line L544 (110.519, -41.6463) -> (110.287, -41.5904)
  line L545 (110.287, -41.5904) -> (110.066, -41.4987)
  line L546 (110.066, -41.4987) -> (109.862, -41.3736)
  line L547 (109.862, -41.3736) -> (109.68, -41.218)
  line L548 (109.68, -41.218) -> (109.524, -41.0358)
  line L549 (109.524, -41.0358) -> (109.4, -40.8316)
  line L550 (109.4, -40.8316) -> (109.308, -40.6104)
  line L551 (109.308, -40.6104) -> (109.253, -40.3776)
  line L552 (109.253, -40.3776) -> (109.236, -40.164)
  line L553 (109.236, -40.164) -> (77.9871, -40.164)
  line L554 (77.9871, -40.164) -> (77.9717, -40.3699)
  line L555 (77.9717, -40.3699) -> (77.9202, -40.5956)
  line L556 (77.9202, -40.5956) -> (77.8356, -40.8111)
  line L557 (77.8356, -40.8111) -> (77.7198, -41.0116)
  line L558 (77.7198, -41.0116) -> (77.5755, -41.1926)
  line L559 (77.5755, -41.1926) -> (77.4058, -41.3501)
  line L560 (77.4058, -41.3501) -> (77.2145, -41.4805)
  line L561 (77.2145, -41.4805) -> (77.0059, -41.5809)
  line L562 (77.0059, -41.5809) -> (76.7847, -41.6492)
  line L563 (76.7847, -41.6492) -> (76.5558, -41.6837)
  line L564 (76.5558, -41.6837) -> (76.3242, -41.6837)
  line L565 (76.3242, -41.6837) -> (76.0953, -41.6492)
  line L566 (76.0953, -41.6492) -> (75.8741, -41.5809)
  line L567 (75.8741, -41.5809) -> (75.6655, -41.4805)
  line L568 (75.6655, -41.4805) -> (75.4742, -41.3501)
  line L569 (75.4742, -41.3501) -> (75.3045, -41.1926)
  line L570 (75.3045, -41.1926) -> (75.1602, -41.0116)
  line L571 (75.1602, -41.0116) -> (75.0444, -40.8111)
  line L572 (75.0444, -40.8111) -> (74.9598, -40.5956)
  line L573 (74.9598, -40.5956) -> (74.9083, -40.3699)
  line L574 (74.9083, -40.3699) -> (74.8929, -40.164)
  line L575 (74.8929, -40.164) -> (43.565, -40.164)
  line L576 (43.565, -40.164) -> (43.5492, -40.3646)
  line L577 (43.5492, -40.3646) -> (43.4963, -40.5847)
  line L578 (43.4963, -40.5847) -> (43.4097, -40.7938)
  line L579 (43.4097, -40.7938) -> (43.2915, -40.9868)
  line L580 (43.2915, -40.9868) -> (43.1445, -41.1589)
  line L581 (43.1445, -41.1589) -> (42.9724, -41.3059)
  line L582 (42.9724, -41.3059) -> (42.7794, -41.4241)
  line L583 (42.7794, -41.4241) -> (42.5703, -41.5107)
  line L584 (42.5703, -41.5107) -> (42.3502, -41.5636)
  line L585 (42.3502, -41.5636) -> (42.1246, -41.5813)
  line L586 (42.1246, -41.5813) -> (41.899, -41.5636)
  line L587 (41.899, -41.5636) -> (41.6789, -41.5107)
  line L588 (41.6789, -41.5107) -> (41.4698, -41.4241)
  line L589 (41.4698, -41.4241) -> (41.2768, -41.3059)
  line L590 (41.2768, -41.3059) -> (41.1047, -41.1589)
  line L591 (41.1047, -41.1589) -> (40.9577, -40.9868)
  line L592 (40.9577, -40.9868) -> (40.8395, -40.7938)
  line L593 (40.8395, -40.7938) -> (40.7529, -40.5847)
  line L594 (40.7529, -40.5847) -> (40.7, -40.3646)
  line L595 (40.7, -40.3646) -> (40.6842, -40.164)
  line L596 (40.6842, -40.164) -> (38.509, -40.164)
  line L597 (38.509, -40.164) -> (38.5086, -40.1638)
  line L598 (38.5086, -40.1638) -> (38.5082, -40.164)
  line L599 (38.5082, -40.164) -> (38.5045, -40.1623)
  line L600 (38.5045, -40.1623) -> (38.4333, -40.1676)
  line L601 (38.4333, -40.1676) -> (38.3611, -40.1888)
  line L602 (38.3611, -40.1888) -> (38.2949, -40.2246)
  line L603 (38.2949, -40.2246) -> (38.2411, -40.2706)
  line L604 (38.2411, -40.2706) -> (38.2392, -40.2752)
  line L605 (38.2392, -40.2752) -> (35.9327, -42.5817)
  line L606 (35.9327, -42.5817) -> (35.9325, -42.5817)
  line L607 (35.9325, -42.5817) -> (35.9325, -42.5819)
  line L608 (35.9325, -42.5819) -> (35.9268, -42.5841)
  line L609 (35.9268, -42.5841) -> (35.8716, -42.6547)
  line L610 (35.8716, -42.6547) -> (35.8346, -42.7425)
  line L611 (35.8346, -42.7425) -> (35.8228, -42.8307)
  line L612 (35.8228, -42.8307) -> (35.825, -42.836)
  line L613 (35.825, -42.836) -> (35.825, -42.837)
  line L614 (35.825, -42.837) -> (35.825, -42.837)
  line L615 (35.825, -42.837) -> (35.825, -42.837)
  line L616 (35.825, -42.837) -> (35.825, -47.4666)
  line L617 (35.825, -47.4666) -> (36.0331, -47.4822)
  line L618 (36.0331, -47.4822) -> (36.2611, -47.5343)
  line L619 (36.2611, -47.5343) -> (36.4787, -47.6197)
  line L620 (36.4787, -47.6197) -> (36.6812, -47.7366)
  line L621 (36.6812, -47.7366) -> (36.864, -47.8823)
  line L622 (36.864, -47.8823) -> (37.023, -48.0537)
  line L623 (37.023, -48.0537) -> (37.1547, -48.2469)
  line L624 (37.1547, -48.2469) -> (37.2561, -48.4575)
  line L625 (37.2561, -48.4575) -> (37.325, -48.6809)
  line L626 (37.325, -48.6809) -> (37.3599, -48.9121)
  line L627 (37.3599, -48.9121) -> (37.3599, -49.1459)
  line L628 (37.3599, -49.1459) -> (37.325, -49.3771)
  line L629 (37.325, -49.3771) -> (37.2561, -49.6005)
  line L630 (37.2561, -49.6005) -> (37.1547, -49.8111)
  line L631 (37.1547, -49.8111) -> (37.023, -50.0043)
  line L632 (37.023, -50.0043) -> (36.864, -50.1757)
  line L633 (36.864, -50.1757) -> (36.6812, -50.3214)
  line L634 (36.6812, -50.3214) -> (36.4787, -50.4383)
  line L635 (36.4787, -50.4383) -> (36.2611, -50.5237)
  line L636 (36.2611, -50.5237) -> (36.0331, -50.5758)
  line L637 (36.0331, -50.5758) -> (35.825, -50.5914)
  line L638 (35.825, -50.5914) -> (35.825, -63.9944)
  line L639 (35.825, -63.9944) -> (36.0305, -64.0098)
  line L640 (36.0305, -64.0098) -> (36.2558, -64.0612)
  line L641 (36.2558, -64.0612) -> (36.471, -64.1457)
  line L642 (36.471, -64.1457) -> (36.6712, -64.2613)
  line L643 (36.6712, -64.2613) -> (36.8519, -64.4054)
  line L644 (36.8519, -64.4054) -> (37.0091, -64.5748)
  line L645 (37.0091, -64.5748) -> (37.1393, -64.7658)
  line L646 (37.1393, -64.7658) -> (37.2396, -64.974)
  line L647 (37.2396, -64.974) -> (37.3077, -65.1949)
  line L648 (37.3077, -65.1949) -> (37.3421, -65.4234)
  line L649 (37.3421, -65.4234) -> (37.3421, -65.6546)
  line L650 (37.3421, -65.6546) -> (37.3077, -65.8831)
  line L651 (37.3077, -65.8831) -> (37.2396, -66.104)
  line L652 (37.2396, -66.104) -> (37.1393, -66.3122)
  line L653 (37.1393, -66.3122) -> (37.0091, -66.5032)
  line L654 (37.0091, -66.5032) -> (36.8519, -66.6726)
  line L655 (36.8519, -66.6726) -> (36.6712, -66.8167)
  line L656 (36.6712, -66.8167) -> (36.471, -66.9323)
  line L657 (36.471, -66.9323) -> (36.2558, -67.0168)
  line L658 (36.2558, -67.0168) -> (36.0305, -67.0682)
  line L659 (36.0305, -67.0682) -> (35.825, -67.0836)
  line L660 (35.825, -67.0836) -> (35.825, -80.4866)
  line L661 (35.825, -80.4866) -> (36.0331, -80.5022)
  line L662 (36.0331, -80.5022) -> (36.2611, -80.5543)
  line L663 (36.2611, -80.5543) -> (36.4787, -80.6397)
  line L664 (36.4787, -80.6397) -> (36.6812, -80.7566)
  line L665 (36.6812, -80.7566) -> (36.864, -80.9023)
  line L666 (36.864, -80.9023) -> (37.023, -81.0737)
  line L667 (37.023, -81.0737) -> (37.1547, -81.2669)
  line L668 (37.1547, -81.2669) -> (37.2561, -81.4775)
  line L669 (37.2561, -81.4775) -> (37.325, -81.7009)
  line L670 (37.325, -81.7009) -> (37.3599, -81.9321)
  line L671 (37.3599, -81.9321) -> (37.3599, -82.1659)
  line L672 (37.3599, -82.1659) -> (37.325, -82.3971)
  line L673 (37.325, -82.3971) -> (37.2561, -82.6205)
  line L674 (37.2561, -82.6205) -> (37.1547, -82.8311)
  line L675 (37.1547, -82.8311) -> (37.023, -83.0243)
  line L676 (37.023, -83.0243) -> (36.864, -83.1957)
  line L677 (36.864, -83.1957) -> (36.6812, -83.3414)
  line L678 (36.6812, -83.3414) -> (36.4787, -83.4583)
  line L679 (36.4787, -83.4583) -> (36.2611, -83.5437)
  line L680 (36.2611, -83.5437) -> (36.0331, -83.5958)
  line L681 (36.0331, -83.5958) -> (35.825, -83.6114)
  line L682 (35.825, -83.6114) -> (35.825, -88.228)
  line L683 (35.825, -88.228) -> (35.8244, -88.2293)
  line L684 (35.8244, -88.2293) -> (35.825, -88.2308)
  line L685 (35.825, -88.2308) -> (35.8233, -88.2345)
  line L686 (35.8233, -88.2345) -> (35.8286, -88.3057)
  line L687 (35.8286, -88.3057) -> (35.8498, -88.3779)
  line L688 (35.8498, -88.3779) -> (35.8856, -88.4441)
  line L689 (35.8856, -88.4441) -> (35.9308, -88.497)
  line L690 (35.9308, -88.497) -> (35.9352, -88.4988)
  line L691 (35.9352, -88.4988) -> (38.2392, -90.8028)
  line L692 (38.2392, -90.8028) -> (38.2411, -90.8075)
  line L693 (38.2411, -90.8075) -> (38.2949, -90.8534)
  line L694 (38.2949, -90.8534) -> (38.3611, -90.8893)
  line L695 (38.3611, -90.8893) -> (38.4333, -90.9104)
  line L696 (38.4333, -90.9104) -> (38.5045, -90.9157)
  line L697 (38.5045, -90.9157) -> (38.5082, -90.914)
  line L698 (38.5082, -90.914) -> (38.5086, -90.9142)
  line L699 (38.5086, -90.9142) -> (38.509, -90.914)
  line L700 (38.509, -90.914) -> (40.5622, -90.914)
  line L701 (40.5622, -90.914) -> (40.5778, -90.7059)
  line L702 (40.5778, -90.7059) -> (40.6299, -90.4779)
  line L703 (40.6299, -90.4779) -> (40.7153, -90.2603)
  line L704 (40.7153, -90.2603) -> (40.8322, -90.0578)
  line L705 (40.8322, -90.0578) -> (40.9779, -89.875)
  line L706 (40.9779, -89.875) -> (41.1493, -89.716)
  line L707 (41.1493, -89.716) -> (41.3425, -89.5843)
  line L708 (41.3425, -89.5843) -> (41.5531, -89.4829)
  line L709 (41.5531, -89.4829) -> (41.7765, -89.414)
  line L710 (41.7765, -89.414) -> (42.0077, -89.3791)
  line L711 (42.0077, -89.3791) -> (42.2415, -89.3791)
  line L712 (42.2415, -89.3791) -> (42.4727, -89.414)
  line L713 (42.4727, -89.414) -> (42.6961, -89.4829)
  line L714 (42.6961, -89.4829) -> (42.9067, -89.5843)
  line L715 (42.9067, -89.5843) -> (43.0999, -89.716)
  line L716 (43.0999, -89.716) -> (43.2713, -89.875)
  line L717 (43.2713, -89.875) -> (43.417, -90.0578)
  line L718 (43.417, -90.0578) -> (43.5339, -90.2603)
  line L719 (43.5339, -90.2603) -> (43.6193, -90.4779)
  line L720 (43.6193, -90.4779) -> (43.6714, -90.7059)
  line L721 (43.6714, -90.7059) -> (43.687, -90.914)
  line L722 (43.687, -90.914) -> (74.8929, -90.914)
  line L723 (74.8929, -90.914) -> (74.9083, -90.7081)
  line L724 (74.9083, -90.7081) -> (74.9598, -90.4824)
  line L725 (74.9598, -90.4824) -> (75.0444, -90.2669)
  line L726 (75.0444, -90.2669) -> (75.1602, -90.0664)
  line L727 (75.1602, -90.0664) -> (75.3045, -89.8854)
  line L728 (75.3045, -89.8854) -> (75.4742, -89.7279)
  line L729 (75.4742, -89.7279) -> (75.6655, -89.5975)
  line L730 (75.6655, -89.5975) -> (75.8741, -89.4971)
  line L731 (75.8741, -89.4971) -> (76.0953, -89.4288)
  line L732 (76.0953, -89.4288) -> (76.3242, -89.3943)
  line L733 (76.3242, -89.3943) -> (76.5558, -89.3943)